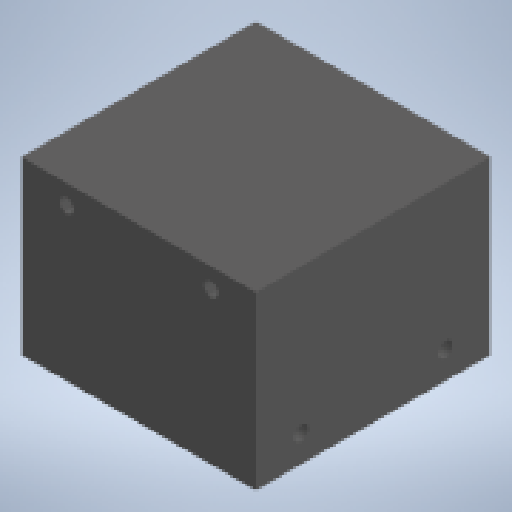
# Autodesk Inventor part: arm_middle
Saved by Autodesk Inventor 2024.1 (Build 281209000, 209)
## iProperties
Created: 2024-02-14
Part Number: arm_middle
Material: 一般
Document SubType Name: Modeling
Designer: hibik
Density: 1 g/cm^3
Appearance: 既定
Author: hibik
Autodesk Inventor part; units mm, degrees
ref_plane "YZ Plane" through (0, 0, 0) normal (1, 0, 0) x (0, 1, 0)
ref_plane "XZ Plane" through (0, 0, 0) normal (0, 1, 0) x (-1, 0, 0)
ref_plane "XY Plane" through (0, 0, 0) normal (0, 0, 1) x (1, 0, 0)
sketch "スケッチ3" plane through (0, 0, 0) normal (1, 0, 0) x (0, 1, 0)
  line L0 (0, 0) -> (4, 0)
  line L1 (4, 0) -> (4, -26)
  line L2 (4, -26) -> (0, -26)
  line L3 (0, -26) -> (0, 0)
  line L4 (4, 0) -> (0, 0)
  line L5 (0, 0) -> (0, -26)
  line L6 (0, -26) -> (4, -26)
  line L7 (4, -26) -> (4, 0)
  line L8 (0, 0) -> (-15, 0)
  line L9 (-15, 0) -> (-15, -26)
  line L10 (-15, -26) -> (0, -26)
  line L11 (0, -26) -> (0, 0)
  dimension "d3" = 26
  dimension "d4" = 4
  dimension "d49" = 15
  constraints: 24 end point, 6 parallel, 3 horizontal, 3 perpendicular, 2 collinear, 1 point on line
  measures "d3" distance of L0.end L1.end
  measures "d4" distance between parallel lines of L1 L5
  measures "d49" distance of L4.end L8.end
extrude "押し出し2" add sketch "スケッチ3" along normal blind 26
sketch "スケッチ10" plane through (26, 0, 0) normal (1, 0, 0) x (0, 0, -1)
  circle A0 centre (5, -12) radius 0.8
  circle A1 centre (21, -12) radius 0.8
  line L0 (0, 4) -> (0, -15) projected
  line L1 (0, -15) -> (26, -15) projected
  point P0 (0, 0)
  dimension "d50" = 1.6
  dimension "d51" = 1.6
  dimension "d52" = 16
  dimension "d53" = 5
  dimension "d54" = 3
  constraints: 2 centre point, 1 horizontal alignment
  measures "d50" diameter of A0
  measures "d51" diameter of A1
  measures "d52" distance of A1.centre A0.centre
  measures "d53" distance from line of L0 A0.centre
  measures "d54" distance from line of L1 A0.centre
extrude "押し出し10" cut sketch "スケッチ10" against normal through all
sketch "スケッチ11" plane through (0, -15, 0) normal (0, 0, 1) x (1, 0, 0)
  circle A0 centre (5, 16.8437) radius 0.8 projected
  circle A1 centre (21, 16.8437) radius 0.8 projected
  point P0 (0, 15)
extrude "押し出し11" cut sketch "スケッチ11" against normal through all
